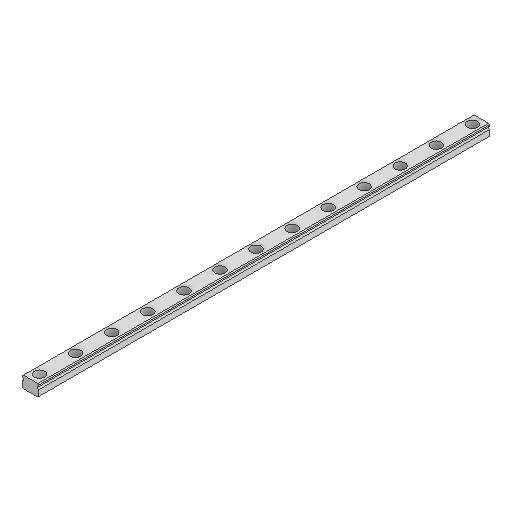
# Autodesk Inventor part: MGNRail250mm
Saved by Autodesk Inventor 2026.2 (Build 302298000, 298)
## iProperties
Created: 2026-03-27
Part Number: MGNRail250mm
Material: Generic
Document SubType Name: Modeling
Designer: gaoet
Density: 1 g/cm^3
Appearance: Default
Author: gaoet
Autodesk Inventor part; units mm, degrees
ref_plane "YZ Plane" through (0, 0, 0) normal (1, 0, 0) x (0, 1, 0)
ref_plane "XZ Plane" through (0, 0, 0) normal (0, 1, 0) x (-1, 0, 0)
ref_plane "XY Plane" through (0, 0, 0) normal (0, 0, 1) x (1, 0, 0)
sketch "Sketch1" plane through (0, 0, 0) normal (0, 0, 1) x (1, 0, 0)
  line L0 (-4.5, -3.25) -> (4.5, -3.25)
  line L1 (4.5, -3.25) -> (4.5, 3.25)
  line L2 (4.5, 3.25) -> (-4.5, 3.25)
  line L3 (-4.5, 3.25) -> (-4.5, -3.25)
  line L4 (-4.5, -3.25) -> (4.5, 3.25) construction
  line L5 (4.5, -3.25) -> (-4.5, 3.25) construction
  circle A0 centre (-4.5, 1.25) radius 0.75
  circle A1 centre (4.5, 1.25) radius 0.75
  line L6 (-3.8126, 0.95) -> (3.8126, 0.95)
  line L7 (3.8126, 0.95) -> (3.8126, 1.55)
  line L8 (3.8126, 1.55) -> (-3.8126, 1.55)
  line L9 (-3.8126, 1.55) -> (-3.8126, 0.95)
  line L10 (-3.8126, 0.95) -> (3.8126, 1.55) construction
  line L11 (3.8126, 0.95) -> (-3.8126, 1.55) construction
  point P0 (0, 0)
  point P1 (0, 1.25)
  point P2 (-4.5, 2)
  point P3 (-4.5, 0.5)
  point P4 (4.5, 0.5)
  point P5 (4.5, 2)
  dimension "d2" = 1.5
  dimension "d0" = 9
  dimension "d1" = 6.5
  dimension "d3" = 4.5
  dimension "d4" = 0.6
  constraints: 24 end point, 4 midpoint, 4 parallel, 2 horizontal, 2 perpendicular, 2 point on circle, 2 vertical alignment, 1 centre point, 1 horizontal alignment, 4 other
  measures "d0" distance of L2.end L1.end
  measures "d1" distance of L1.end L0.end
  measures "d3" distance from line of L0 point (-4.5, 1.25)
  measures "d4" distance of L6.end L7.end
extrude "Extrusion1" add sketch "Sketch1" along normal blind 250 contours L3 A0 L6 A1 L1 L0 | L3 L2 L1 A1 L8 A0 | A0 L8 A1 L6
chamfer "Chamfer1" distance 0.5 angle 45 4 edges at (-4.5, 3.25, 125) (-4.5, -3.25, 125) (4.5, 3.25, 125) (4.5, -3.25, 125)
sketch "Sketch2" plane through (-4, 3.25, 0) normal (0, 1, 0) x (1, 0, 0)
  line L0 (-0.5, 0) -> (-0.5, -250) projected
  line L1 (8, 0) -> (0, 0) projected
  point P0 (4, 0)
  point P1 (4, -5)
  point P2 (4, -25)
  point P3 (4, -45)
  point P4 (4, -65)
  point P5 (4, -85)
  point P6 (4, -105)
  point P7 (4, -125)
  point P8 (4, -145)
  point P9 (4, -165)
  point P10 (4, -185)
  point P11 (4, -205)
  point P12 (4, -225)
  point P13 (4, -245)
  dimension "d10" = 4.5
  dimension "d13" = 20
  dimension "d18" = 5
  constraints: 1 vertical, 12 other
  measures "d10" distance from line of L0 point (4, -5)
  measures "d13" distance of point (4, -5) point (4, -25)
  measures "d18" distance from line of L1 point (4, -5)
hole "Hole1" at (0, 3.25, 5) at (0, 3.25, 25) at (0, 3.25, 45) at (0, 3.25, 65) at (0, 3.25, 85) at (0, 3.25, 105) at (0, 3.25, 125) at (0, 3.25, 145) at (0, 3.25, 165) at (0, 3.25, 185) at (0, 3.25, 205) at (0, 3.25, 225) at (0, 3.25, 245) direction (0, -1, 0) diameter 3.3 depth 10 counterbore diameter 5.7 counterbore depth 4
body "Solid1"
